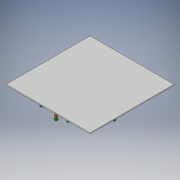
# Autodesk Inventor part: parker
Saved by Autodesk Inventor 2018 (Build 220112000, 112)
## iProperties
Created: 2018-06-06
Part Number: parker
Material: Generic
Document SubType Name: Modeling
Designer: 3400746
Density: 1 g/cm^3
Appearance: Default
Author: 3400746
Autodesk Inventor part; units mm, degrees
sketch "Sketch1" plane through (0, 0, 0) normal (0, 1, 0) x (-1, 0, 0)
  line L0 (0, 0) -> (-2159, 0)
  line L1 (-2159, 0) -> (-2159, 2159)
  line L2 (-2159, 2159) -> (0, 2159)
  line L3 (0, 2159) -> (0, 0)
  dimension "d0" = 2159
  dimension "d1" = 2159
  dimension "d2" = 2159
  constraints: 8 end point, 2 perpendicular, 1 horizontal
  measures "d0" distance of L0.start L0.end
  measures "d1" distance of L0.end L1.end
  measures "d2" distance of L1.end L2.end
extrude "Extrusion1" add sketch "Sketch1" against normal blind 25.4
sketch "Sketch2" plane through (0, -25.4, 0) normal (0, -1, 0) x (1, 0, 0)
  line L0 (0, 0) -> (0, 1079.5)
  line L1 (0, 2159) -> (0, 0) projected
  line L2 (0, 1079.5) -> (0, 1016)
  line L3 (0, 1079.5) -> (0, 1143)
  line L4 (2159, 0) -> (2159, 2159) projected
  line L5 (0, 0) -> (2159, 0) projected
  line L6 (0, 0) -> (1079.5, 0)
  line L7 (1079.5, 0) -> (1143, 0)
  line L8 (1079.5, 0) -> (1016, 0)
  line L9 (0, 1016) -> (1016, 1016)
  line L10 (1016, 0) -> (1016, 1016)
  line L11 (1016, 0) -> (1143, 0)
  line L12 (1143, 0) -> (1143, 1016)
  line L13 (1143, 1016) -> (2159, 1016)
  line L14 (2159, 1016) -> (2159, 1143)
  line L15 (2159, 1143) -> (1143, 1143)
  line L16 (1143, 1143) -> (1143, 2159)
  line L17 (1143, 2159) -> (1016, 2159)
  line L18 (2159, 2159) -> (0, 2159) projected
  line L19 (1016, 2159) -> (1016, 1143)
  line L20 (1016, 1143) -> (0, 1143)
  line L21 (0, 1143) -> (0, 1016)
  dimension "d5" = 63.5
  dimension "d6" = 63.5
  dimension "d7" = 1079.5
  dimension "d8" = 63.5
  dimension "d9" = 63.5
  constraints: 36 end point, 6 point on line, 3 perpendicular, 2 collinear, 1 midpoint
  measures "d5" distance of L0.end L2.end
  measures "d6" distance of L0.end L3.end
  measures "d7" distance of L0.start L6.end
  measures "d8" distance of L6.end L7.end
  measures "d9" distance of L6.end L8.end
extrude "Extrusion2" add sketch "Sketch2" along normal blind 2.54 contours L0 L1 L20 L19 L17 L16 L15 L4 L13 L12 L5 L10 L9
sketch "Sketch3" plane through (0, -25.4, 0) normal (0, -1, 0) x (1, 0, 0)
  line L0 (0, 2159) -> (0, 0) projected
  line L1 (0, 0) -> (0, 539.75)
  line L2 (0, 539.75) -> (508, 539.75)
  line L3 (508, 539.75) -> (508, 0)
  line L4 (508, 539.75) -> (508, 777.875)
  line L5 (508, 777.875) -> (762, 777.875)
  circle A0 centre (762, 777.875) radius 38.1
  line L6 (508, 269.875) -> (254, 269.875)
  circle A1 centre (254, 269.875) radius 35.56
  line L7 (508, 539.75) -> (818.4812, 539.75)
  circle A2 centre (818.4812, 539.75) radius 25.4
  line L8 (64.4175, 539.75) -> (64.4175, 939.7377)
  circle A3 centre (64.4175, 939.7377) radius 31.75
  line L9 (508, 115.5726) -> (863.9524, 246.3022)
  circle A4 centre (863.9524, 246.3022) radius 29.21
  line L10 (316.4036, 539.75) -> (286.0895, 847.725)
  circle A5 centre (286.0895, 847.725) radius 25.4
  line L11 (508, 539.75) -> (557.9761, 607.8668)
  circle A6 centre (557.9761, 607.8668) radius 31.75
  line L12 (2158.5018, 0) -> (1618.7518, 0)
  line L13 (1618.7518, 0) -> (1618.7518, 508)
  line L14 (1618.7518, 508) -> (2158.5018, 508)
  line L15 (1618.7518, 508) -> (1380.6268, 508)
  circle A7 centre (1380.6268, 762) radius 38.1
  line L16 (1888.6268, 508) -> (1888.6268, 254)
  circle A8 centre (1888.6268, 254) radius 35.56
  circle A9 centre (1618.7518, 818.4812) radius 25.4
  line L17 (1618.7518, 64.4175) -> (1218.7641, 64.4175)
  circle A10 centre (1218.7641, 64.4175) radius 31.75
  line L18 (2042.9293, 508) -> (1912.1996, 863.9524)
  circle A11 centre (1912.1996, 863.9524) radius 29.21
  line L19 (1618.7518, 316.4036) -> (1310.7768, 286.0895)
  circle A12 centre (1310.7768, 286.0895) radius 25.4
  circle A13 centre (1550.635, 557.9761) radius 31.75
  line L20 (0, 1146.7792) -> (0, 1686.5292)
  line L21 (472.4708, 1146.7792) -> (472.4708, 1654.7792)
  line L22 (472.4708, 1654.7792) -> (1012.2208, 1654.7792)
  line L23 (472.4708, 1654.7792) -> (234.3458, 1654.7792)
  circle A14 centre (234.3458, 1908.7792) radius 38.1
  line L24 (742.3458, 1654.7792) -> (742.3458, 1400.7792)
  circle A15 centre (742.3458, 1400.7792) radius 35.56
  circle A16 centre (472.4708, 1965.2604) radius 25.4
  line L25 (472.4708, 1211.1967) -> (72.4831, 1211.1967)
  circle A17 centre (72.4831, 1211.1967) radius 31.75
  line L26 (896.6483, 1654.7792) -> (765.9186, 2010.7316)
  circle A18 centre (765.9186, 2010.7316) radius 29.21
  line L27 (472.4708, 1463.1828) -> (164.4958, 1432.8687)
  circle A19 centre (164.4958, 1432.8687) radius 25.4
  circle A20 centre (404.354, 1704.7553) radius 31.75
  line L28 (1145.3553, 1146.7792) -> (1145.3553, 1686.5292)
  line L29 (1145.3553, 1686.5292) -> (1653.3553, 1686.5292)
  line L30 (1653.3553, 1686.5292) -> (1653.3553, 1146.7792)
  line L31 (1653.3553, 1686.5292) -> (1653.3553, 1924.6542)
  circle A21 centre (1907.3553, 1924.6542) radius 38.1
  line L32 (1653.3553, 1416.6542) -> (1399.3553, 1416.6542)
  circle A22 centre (1399.3553, 1416.6542) radius 35.56
  circle A23 centre (1963.8365, 1686.5292) radius 25.4
  line L33 (1209.7728, 1686.5292) -> (1209.7728, 2086.5169)
  circle A24 centre (1209.7728, 2086.5169) radius 31.75
  line L34 (1653.3553, 1262.3517) -> (2009.3077, 1393.0814)
  circle A25 centre (2009.3077, 1393.0814) radius 29.21
  line L35 (1461.7589, 1686.5292) -> (1431.4448, 1994.5042)
  circle A26 centre (1431.4448, 1994.5042) radius 25.4
  circle A27 centre (1703.3314, 1754.646) radius 31.75
  dimension "d12" = 539.75
  dimension "d13" = 508
  dimension "d14" = 238.125
  dimension "d15" = 254
  dimension "d16" = 76.2
  dimension "d17" = 254
  dimension "d18" = 71.12
  dimension "d19" = 50.8
  dimension "d20" = 63.5
  dimension "d21" = 58.42
  dimension "d22" = 50.8
  dimension "d67" = 63.5
  dimension "d74" = 539.75
  dimension "d75" = 508
  dimension "d76" = 238.125
  dimension "d77" = 76.2
  dimension "d78" = 254
  dimension "d79" = 71.12
  dimension "d80" = 50.8
  dimension "d81" = 63.5
  dimension "d82" = 58.42
  dimension "d83" = 50.8
  dimension "d84" = 63.5
  dimension "d85" = 539.75
  dimension "d86" = 508
  dimension "d87" = 238.125
  dimension "d88" = 76.2
  dimension "d89" = 254
  dimension "d90" = 71.12
  dimension "d91" = 50.8
  dimension "d92" = 63.5
  dimension "d93" = 58.42
  dimension "d94" = 50.8
  dimension "d95" = 63.5
  dimension "d96" = 539.75
  dimension "d97" = 508
  dimension "d98" = 238.125
  dimension "d99" = 76.2
  dimension "d100" = 254
  dimension "d101" = 71.12
  dimension "d102" = 50.8
  dimension "d103" = 63.5
  dimension "d104" = 58.42
  dimension "d105" = 50.8
  dimension "d106" = 63.5
  constraints: 70 end point, 28 centre point, 19 coincident, 13 point on line, 8 perpendicular, 4 midpoint, 4 vertical, 3 horizontal
  measures "d12" distance of L0.end L1.end
  measures "d13" distance of L1.end L2.end
  measures "d14" distance of L2.end L4.end
  measures "d15" distance of L4.end L5.end
  measures "d16" diameter of A0
  measures "d17" distance of L6.start L6.end
  measures "d18" diameter of A1
  measures "d19" diameter of A2
  measures "d20" diameter of A3
  measures "d21" diameter of A4
  measures "d22" diameter of A5
  measures "d67" diameter of A6
  measures "d74" distance of L12.start L13.start
  measures "d75" distance of L13.start L13.end
  measures "d76" distance of L13.end L15.end
  measures "d77" diameter of A7
  measures "d78" distance of L16.start L16.end
  measures "d79" diameter of A8
  measures "d80" diameter of A9
  measures "d81" diameter of A10
  measures "d82" diameter of A11
  measures "d83" diameter of A12
  measures "d84" diameter of A13
  measures "d85" distance of L20.end L20.start
  measures "d86" distance of L21.start L21.end
  measures "d87" distance of L21.end L23.end
  measures "d88" diameter of A14
  measures "d89" distance of L24.start L24.end
  measures "d90" diameter of A15
  measures "d91" diameter of A16
  measures "d92" diameter of A17
  measures "d93" diameter of A18
  measures "d94" diameter of A19
  measures "d95" diameter of A20
  measures "d96" distance of L28.start L29.start
  measures "d97" distance of L29.start L29.end
  measures "d98" distance of L29.end L31.end
  measures "d99" diameter of A21
  measures "d100" distance of L32.start L32.end
  measures "d101" diameter of A22
  measures "d102" diameter of A23
  measures "d103" diameter of A24
  measures "d104" diameter of A25
  measures "d105" diameter of A26
  measures "d106" diameter of A27
extrude "Extrusion5" add sketch "Sketch3" along normal blind 127 contours A0
extrude "Extrusion6" add sketch "Sketch3" along normal blind 152.4 contours A2
extrude "Extrusion7" add sketch "Sketch3" along normal blind 127 contours A4
extrude "Extrusion8" add sketch "Sketch3" along normal blind 165.1 contours A1
extrude "Extrusion9" add sketch "Sketch3" along normal blind 152.4 contours A5
extrude "Extrusion10" add sketch "Sketch3" along normal blind 177.8 contours A3
ref_plane "Work Plane1" through (64.4175, -203.2, 907.9877) normal (1, 0, 0) x (0, 0, 1)
sketch "Sketch10" plane through (64.4175, -203.2, 907.9877) normal (1, 0, 0) x (0, 0, 1)
  line L0 (63.5, 0) -> (0, 0) projected
  line L1 (31.75, 0) -> (31.75, 50.9666)
  line L2 (31.75, 0) -> (31.75, -50.9778)
  arc A0 (31.75, 50.9666) -> (31.75, -50.9778) centre (16.1162, -0.0056) ccw
  point P0 (-907.9877, -203.2)
  dimension "d41" = 50.9778
  constraints: 4 end point, 2 point on circle, 2 vertical, 1 centre point, 1 midpoint
  measures "d41" distance of L1.start L2.end
sketch "Sketch11" plane through (286.0895, -177.8, 847.725) normal (0, -1, 0) x (1, 0, 0)
  line L0 (0, 0) -> (0, -25.4)
  circle A0 centre (0, 0) radius 25.4 projected
  point P0 (-286.0895, -847.725)
  constraints: 2 end point, 1 vertical, 1 vertical alignment, 1 other
ref_plane "Work Plane2" through (286.0895, -177.8, 847.725) normal (-1, 0, 0) x (0, 0, -1)
sketch "Sketch12" plane through (286.0895, -177.8, 847.725) normal (-1, 0, 0) x (0, 0, -1)
  line L0 (25.4, 0) -> (-25.4, 0) projected
  line L1 (0, 0) -> (0, 45.72)
  line L2 (0, 0) -> (0, -45.72)
  arc A0 (0, -45.72) -> (0, 45.72) centre (5.3528, 0) ccw
  point P0 (847.725, -177.8)
  dimension "d44" = 45.72
  dimension "d45" = 45.72
  constraints: 4 end point, 2 point on circle, 2 vertical, 1 centre point, 1 midpoint
  measures "d44" distance of L1.start L1.end
  measures "d45" distance of L1.start L2.end
revolve "Revolution2" add sketch "Sketch12" angle 360 about axis through (286.0895, -177.8, 847.725) along (0, -1, 0)
revolve "Revolution3" add sketch "Sketch10" angle 360 about axis through (64.4175, -203.2, 939.7377) along (0, -1, 0)
sketch "Sketch13" plane through (762, -152.4, 777.875) normal (0, -1, 0) x (1, 0, 0)
  line L0 (0, 0) -> (0, -38.1)
  circle A0 centre (0, 0) radius 38.1 projected
  point P0 (-762, -777.875)
  constraints: 2 end point, 1 vertical, 1 vertical alignment, 1 other
ref_plane "Work Plane3" through (762, -152.4, 777.875) normal (-1, 0, 0) x (0, 0, -1)
sketch "Sketch14" plane through (762, -152.4, 777.875) normal (-1, 0, 0) x (0, 0, -1)
  line L0 (38.1, 0) -> (-38.1, 0) projected
  line L1 (0, 0) -> (0, 53.34)
  line L2 (0, 0) -> (0, -53.34)
  arc A0 (0, -53.34) -> (0, 53.34) centre (4.894, 0) ccw
  point P0 (777.875, -152.4)
  dimension "d49" = 53.34
  dimension "d50" = 53.34
  constraints: 4 end point, 2 point on circle, 2 vertical, 1 centre point, 1 midpoint
  measures "d49" distance of L1.start L1.end
  measures "d50" distance of L1.start L2.end
revolve "Revolution4" add sketch "Sketch14" angle 360 about axis through (762, -152.4, 777.875) along (0, -1, 0)
sketch "Sketch15" plane through (818.4812, -177.8, 539.75) normal (0, -1, 0) x (1, 0, 0)
  line L0 (0, 0) -> (0, -25.4)
  circle A0 centre (0, 0) radius 25.4 projected
  point P0 (-818.4812, -539.75)
  constraints: 2 end point, 1 vertical, 1 vertical alignment, 1 other
ref_plane "Work Plane4" through (818.4812, -177.8, 539.75) normal (-1, 0, 0) x (0, 0, -1)
sketch "Sketch17" plane through (818.4812, -177.8, 539.75) normal (-1, 0, 0) x (0, 0, -1)
  line L0 (25.4, 0) -> (-25.4, 0) projected
  line L1 (0, 0) -> (0, 43.18)
  line L2 (0, 0) -> (0, -43.18)
  arc A0 (0, -43.18) -> (0, 43.18) centre (-0.7299, 0) ccw
  point P0 (539.75, -177.8)
  dimension "d53" = 43.18
  dimension "d54" = 43.18
  constraints: 4 end point, 2 point on circle, 2 vertical, 1 centre point, 1 midpoint
  measures "d53" distance of L1.start L1.end
  measures "d54" distance of L1.start L2.end
revolve "Revolution5" add sketch "Sketch17" angle 360 about axis through (818.4812, -177.8, 539.75) along (0, -1, 0)
sketch "Sketch18" plane through (863.9524, -152.4, 246.3022) normal (0, -1, 0) x (1, 0, 0)
  circle A0 centre (0, 0) radius 29.21 projected
  line L0 (0, 0) -> (0, -29.21)
  point P0 (-863.9524, -246.3022)
  constraints: 2 end point, 1 vertical, 1 vertical alignment, 1 other
ref_plane "Work Plane5" through (863.9524, -152.4, 246.3022) normal (-1, 0, 0) x (0, 0, -1)
sketch "Sketch19" plane through (863.9524, -152.4, 246.3022) normal (-1, 0, 0) x (0, 0, -1)
  line L0 (29.21, 0) -> (-29.21, 0) projected
  line L1 (0, 0) -> (0, 38.1)
  line L2 (0, 0) -> (0, -38.1)
  arc A0 (0, -38.1) -> (0, 38.1) centre (14.1421, 0) ccw
  point P0 (246.3022, -152.4)
  dimension "d57" = 38.1
  dimension "d58" = 38.1
  dimension "d59" = 40.64
  constraints: 4 end point, 2 point on circle, 2 vertical, 1 centre point, 1 midpoint
  measures "d57" distance of L1.start L1.end
  measures "d58" distance of L1.start L2.end
  measures "d59" radius of A0
revolve "Revolution6" add sketch "Sketch19" angle 360 about axis through (863.9524, -152.4, 246.3022) along (0, -1, 0)
sketch "Sketch20" plane through (254, -190.5, 269.875) normal (0, -1, 0) x (1, 0, 0)
  line L0 (0, 0) -> (0, -35.56)
  circle A0 centre (0, 0) radius 35.56 projected
  point P0 (-254, -269.875)
  constraints: 2 end point, 1 vertical, 1 vertical alignment, 1 other
ref_plane "Work Plane6" through (254, -190.5, 269.875) normal (-1, 0, 0) x (0, 0, -1)
sketch "Sketch21" plane through (254, -190.5, 269.875) normal (-1, 0, 0) x (0, 0, -1)
  line L0 (35.56, 0) -> (-35.56, 0) projected
  line L1 (0, 0) -> (0, 55.88)
  line L2 (0, 0) -> (0, -55.88)
  arc A0 (0, -55.88) -> (0, 55.88) centre (11.9812, 0) ccw
  point P0 (269.875, -190.5)
  dimension "d63" = 55.88
  dimension "d64" = 55.88
  dimension "d65" = 57.15
  constraints: 4 end point, 2 point on circle, 2 vertical, 1 centre point, 1 midpoint
  measures "d63" distance of L1.start L1.end
  measures "d64" distance of L1.start L2.end
  measures "d65" radius of A0
revolve "Revolution7" add sketch "Sketch21" angle 360 about axis through (254, -190.5, 269.875) along (0, -1, 0)
extrude "Extrusion11" add sketch "Sketch3" along normal blind 139.7 contours A6
sketch "Sketch22" plane through (557.9761, -165.1, 607.8668) normal (0, -1, 0) x (1, 0, 0)
  line L0 (0, 0) -> (0, -31.75)
  circle A0 centre (0, 0) radius 31.75 projected
  point P0 (-557.9761, -607.8668)
  constraints: 2 end point, 1 vertical, 1 vertical alignment, 1 other
ref_plane "Work Plane7" through (557.9761, -165.1, 607.8668) normal (-1, 0, 0) x (0, 0, -1)
sketch "Sketch23" plane through (557.9761, -165.1, 607.8668) normal (-1, 0, 0) x (0, 0, -1)
  line L0 (31.75, 0) -> (-31.75, 0) projected
  line L1 (0, 0) -> (0, 48.26)
  line L2 (0, 0) -> (0, -48.26)
  arc A0 (0, -48.26) -> (0, 48.26) centre (-0.8159, 0) ccw
  point P0 (607.8668, -165.1)
  dimension "d71" = 48.26
  dimension "d72" = 48.26
  constraints: 4 end point, 2 point on circle, 2 vertical, 1 centre point, 1 midpoint
  measures "d71" distance of L1.start L1.end
  measures "d72" distance of L1.start L2.end
revolve "Revolution8" add sketch "Sketch23" angle 360 about axis through (557.9761, -165.1, 607.8668) along (0, -1, 0)
extrude "Extrusion12" add sketch "Sketch3" along normal blind 127 contours A7 | A15 | A22
sketch "Sketch24" plane through (1399.3553, -152.4, 1416.6542) normal (0, -1, 0) x (1, 0, 0)
  line L0 (0, 0) -> (0, -35.56)
  circle A0 centre (0, 0) radius 35.56 projected
  point P0 (-1399.3553, -1416.6542)
  constraints: 2 end point, 1 vertical, 1 vertical alignment, 1 other
ref_plane "Work Plane8" through (1399.3553, -152.4, 1416.6542) normal (-1, 0, 0) x (0, 0, -1)
sketch "Sketch25" plane through (1399.3553, -152.4, 1416.6542) normal (-1, 0, 0) x (0, 0, -1)
  line L0 (0, 0) -> (0, 50.8)
  line L1 (0, 0) -> (0, -50.8)
  arc A0 (0, -50.8) -> (0, 50.8) centre (0, 0) ccw
  point P0 (1416.6542, -152.4)
  dimension "d110" = 50.8
  dimension "d111" = 50.8
  dimension "d112" = 50.8
  constraints: 4 end point, 2 point on circle, 2 vertical, 1 centre point
  measures "d110" distance of L0.start L0.end
  measures "d111" distance of L0.start L1.end
  measures "d112" radius of A0
revolve "Revolution9" add sketch "Sketch25" angle 360 about axis through (1399.3553, -152.4, 1416.6542) along (0, -1, 0)
sketch "Sketch26" plane through (1380.6268, -152.4, 762) normal (0, -1, 0) x (1, 0, 0)
  line L0 (0, 0) -> (0, -38.1)
  circle A0 centre (0, 0) radius 38.1 projected
  point P0 (-1380.6268, -762)
  constraints: 2 end point, 1 vertical, 1 vertical alignment, 1 other
ref_plane "Work Plane9" through (1380.6268, -152.4, 762) normal (-1, 0, 0) x (0, 0, -1)
sketch "Sketch27" plane through (1380.6268, -152.4, 762) normal (-1, 0, 0) x (0, 0, -1)
  line L0 (38.1, 0) -> (-38.1, 0) projected
  line L1 (0, 0) -> (0, 50.8)
  line L2 (0, 0) -> (0, -50.8)
  arc A0 (0, -50.8) -> (0, 50.8) centre (0, 0) ccw
  point P0 (762, -152.4)
  dimension "d115" = 50.8
  dimension "d116" = 50.8
  dimension "d117" = 50.8
  constraints: 4 end point, 2 point on circle, 2 vertical, 1 centre point, 1 midpoint
  measures "d115" distance of L1.start L1.end
  measures "d116" distance of L1.start L2.end
  measures "d117" radius of A0
revolve "Revolution10" add sketch "Sketch27" angle 360 about axis through (1380.6268, -152.4, 762) along (0, -1, 0)
sketch "Sketch28" plane through (742.3458, -152.4, 1400.7792) normal (0, -1, 0) x (1, 0, 0)
  circle A0 centre (0, 0) radius 35.56 projected
  line L0 (0, 0) -> (0, -35.56)
  point P0 (-742.3458, -1400.7792)
  constraints: 2 end point, 1 vertical, 1 vertical alignment, 1 other
ref_plane "Work Plane10" through (742.3458, -152.4, 1400.7792) normal (-1, 0, 0) x (0, 0, -1)
sketch "Sketch29" plane through (742.3458, -152.4, 1400.7792) normal (-1, 0, 0) x (0, 0, -1)
  line L0 (0, 0) -> (0, 50.8)
  line L1 (0, 0) -> (0, -50.8)
  arc A0 (0, -50.8) -> (0, 50.8) centre (0, 0) ccw
  point P0 (1400.7792, -152.4)
  dimension "d120" = 50.8
  dimension "d121" = 50.8
  dimension "d122" = 50.8
  constraints: 4 end point, 2 point on circle, 2 vertical, 1 centre point
  measures "d120" distance of L0.start L0.end
  measures "d121" distance of L0.start L1.end
  measures "d122" radius of A0
revolve "Revolution11" add sketch "Sketch29" angle 360 about axis through (742.3458, -152.4, 1400.7792) along (0, -1, 0)
extrude "Extrusion13" add sketch "Sketch3" along normal blind 127 contours A11 | A18 | A25
sketch "Sketch30" plane through (765.9186, -152.4, 2010.7316) normal (0, -1, 0) x (1, 0, 0)
  circle A0 centre (0, 0) radius 29.21 projected
  line L0 (0, 0) -> (0, -38.1)
  point P0 (-765.9186, -2010.7316)
  dimension "d126" = 38.1
  constraints: 2 end point, 1 vertical
  measures "d126" distance of L0.start L0.end
ref_plane "Work Plane11" through (765.9186, -152.4, 2010.7316) normal (-1, 0, 0) x (0, 0, -1)
sketch "Sketch31" plane through (765.9186, -152.4, 2010.7316) normal (-1, 0, 0) x (0, 0, -1)
  line L0 (0, 0) -> (0, 45.72)
  line L1 (0, 0) -> (0, -45.72)
  arc A0 (0, -45.72) -> (0, 45.72) centre (0, 0) ccw
  point P0 (2010.7316, -152.4)
  dimension "d128" = 45.72
  dimension "d129" = 45.72
  dimension "d130" = 45.72
  constraints: 4 end point, 2 point on circle, 2 vertical, 1 centre point
  measures "d128" distance of L0.start L0.end
  measures "d129" distance of L0.start L1.end
  measures "d130" radius of A0
revolve "Revolution12" add sketch "Sketch31" angle 360 about axis through (765.9186, -152.4, 2010.7316) along (0, -1, 0)
sketch "Sketch32" plane through (2009.3077, -152.4, 1393.0814) normal (0, -1, 0) x (1, 0, 0)
  line L0 (0, 0) -> (0, -29.21)
  circle A0 centre (0, 0) radius 29.21 projected
  point P0 (-2009.3077, -1393.0814)
  constraints: 2 end point, 1 vertical, 1 vertical alignment, 1 other
ref_plane "Work Plane12" through (2009.3077, -152.4, 1393.0814) normal (-1, 0, 0) x (0, 0, -1)
sketch "Sketch33" plane through (2009.3077, -152.4, 1393.0814) normal (-1, 0, 0) x (0, 0, -1)
  line L0 (0, 0) -> (0, 45.72)
  line L1 (0, 0) -> (0, -45.72)
  arc A0 (0, -45.72) -> (0, 45.72) centre (0, 0) ccw
  point P0 (1393.0814, -152.4)
  dimension "d133" = 45.72
  dimension "d134" = 45.72
  dimension "d135" = 45.72
  constraints: 4 end point, 2 point on circle, 2 vertical, 1 centre point
  measures "d133" distance of L0.start L0.end
  measures "d134" distance of L0.start L1.end
  measures "d135" radius of A0
revolve "Revolution13" add sketch "Sketch33" angle 360 about axis through (2009.3077, -152.4, 1393.0814) along (0, -1, 0)
sketch "Sketch34" plane through (1912.1996, -152.4, 863.9524) normal (0, -1, 0) x (1, 0, 0)
  line L0 (0, 0) -> (0, -29.21)
  circle A0 centre (0, 0) radius 29.21 projected
  point P0 (-1912.1996, -863.9524)
  constraints: 2 end point, 1 vertical, 1 vertical alignment, 1 other
ref_plane "Work Plane13" through (1912.1996, -152.4, 863.9524) normal (-1, 0, 0) x (0, 0, -1)
sketch "Sketch35" plane through (1912.1996, -152.4, 863.9524) normal (-1, 0, 0) x (0, 0, -1)
  line L0 (0, 0) -> (0, 45.72)
  line L1 (0, 0) -> (0, -45.72)
  arc A0 (0, -45.72) -> (0, 45.72) centre (0, 0) ccw
  point P0 (863.9524, -152.4)
  dimension "d138" = 45.72
  dimension "d140" = 45.72
  dimension "d141" = 45.72
  constraints: 4 end point, 2 point on circle, 2 vertical, 1 centre point
  measures "d138" distance of L0.start L0.end
  measures "d140" distance of L0.start L1.end
  measures "d141" radius of A0
revolve "Revolution14" add sketch "Sketch35" angle 360 about axis through (1912.1996, -152.4, 863.9524) along (0, -1, 0)
extrude "Extrusion14" add sketch "Sketch3" along normal blind 152.4 contours A9 | A12 | A16 | A19 | A23 | A26
sketch "Sketch36" plane through (472.4708, -177.8, 1965.2604) normal (0, -1, 0) x (1, 0, 0)
  circle A0 centre (0, 0) radius 25.4 projected
  line L0 (0, 0) -> (0, -25.4)
  point P0 (-472.4708, -1965.2604)
  constraints: 2 end point, 1 vertical, 1 vertical alignment, 1 other
ref_plane "Work Plane14" through (472.4708, -177.8, 1965.2604) normal (-1, 0, 0) x (0, 0, -1)
sketch "Sketch37" plane through (472.4708, -177.8, 1965.2604) normal (-1, 0, 0) x (0, 0, -1)
  line L0 (0, 0) -> (0, 38.1)
  line L1 (0, 0) -> (0, -38.1)
  arc A0 (0, -38.1) -> (0, 38.1) centre (0, 0) ccw
  point P0 (1965.2604, -177.8)
  dimension "d146" = 38.1
  dimension "d147" = 38.1
  dimension "d148" = 38.1
  constraints: 4 end point, 2 point on circle, 2 vertical, 1 centre point
  measures "d146" distance of L0.start L0.end
  measures "d147" distance of L0.start L1.end
  measures "d148" radius of A0
revolve "Revolution15" add sketch "Sketch37" angle 360 about axis through (472.4708, -177.8, 1965.2604) along (0, -1, 0)
sketch "Sketch38" plane through (164.4958, -177.8, 1432.8687) normal (0, -1, 0) x (1, 0, 0)
  circle A0 centre (0, 0) radius 25.4 projected
  line L0 (0, 0) -> (0, -25.4)
  point P0 (-164.4958, -1432.8687)
  constraints: 2 end point, 1 vertical, 1 vertical alignment, 1 other
ref_plane "Work Plane15" through (164.4958, -177.8, 1432.8687) normal (-1, 0, 0) x (0, 0, -1)
sketch "Sketch39" plane through (164.4958, -177.8, 1432.8687) normal (-1, 0, 0) x (0, 0, -1)
  line L0 (25.4, 0) -> (-25.4, 0) projected
  line L1 (0, 0) -> (0, 38.1)
  line L2 (0, 0) -> (0, -38.1)
  arc A0 (0, -38.1) -> (0, 38.1) centre (0, 0) ccw
  point P0 (1432.8687, -177.8)
  dimension "d151" = 38.1
  dimension "d152" = 38.1
  dimension "d153" = 38.1
  constraints: 4 end point, 2 point on circle, 2 vertical, 1 centre point, 1 midpoint
  measures "d151" distance of L1.start L1.end
  measures "d152" distance of L1.start L2.end
  measures "d153" radius of A0
revolve "Revolution16" add sketch "Sketch39" angle 360 about axis through (164.4958, -177.8, 1432.8687) along (0, -1, 0)
sketch "Sketch40" plane through (1431.4448, -177.8, 1994.5042) normal (0, -1, 0) x (1, 0, 0)
  line L0 (0, 0) -> (0, -25.5263)
  point P0 (-1431.4448, -1994.5042)
  constraints: 2 end point, 1 vertical
ref_plane "Work Plane16" through (1431.4448, -177.8, 1994.5042) normal (-1, 0, 0) x (0, 0, -1)
sketch "Sketch41" plane through (1431.4448, -177.8, 1994.5042) normal (-1, 0, 0) x (0, 0, -1)
  line L0 (0, 0) -> (0, 38.1)
  line L1 (0, 0) -> (0, -38.1)
  arc A0 (0, -38.1) -> (0, 38.1) centre (0, 0) ccw
  point P0 (1994.5042, -177.8)
  dimension "d156" = 38.1
  dimension "d158" = 38.1
  dimension "d159" = 38.1
  constraints: 4 end point, 2 point on circle, 1 centre point, 1 point on line, 1 vertical
  measures "d156" distance of L0.start L0.end
  measures "d158" distance of L0.start L1.end
  measures "d159" radius of A0
revolve "Revolution17" add sketch "Sketch41" angle 360 about axis through (1431.4448, -177.8, 1994.5042) along (0, -1, 0)
sketch "Sketch42" plane through (1963.8365, -177.8, 1686.5292) normal (0, -1, 0) x (1, 0, 0)
  line L0 (0, 0) -> (0, -25.4)
  circle A0 centre (0, 0) radius 25.4 projected
  point P0 (-1963.8365, -1686.5292)
  constraints: 2 end point, 1 vertical, 1 vertical alignment, 1 other
ref_plane "Work Plane17" through (1963.8365, -177.8, 1686.5292) normal (-1, 0, 0) x (0, 0, -1)
sketch "Sketch43" plane through (1963.8365, -177.8, 1686.5292) normal (-1, 0, 0) x (0, 0, -1)
  line L0 (25.4, 0) -> (-25.4, 0) projected
  line L1 (0, 0) -> (0, 38.1)
  line L2 (0, 0) -> (0, -38.1)
  arc A0 (0, -38.1) -> (0, 38.1) centre (0, 0) ccw
  point P0 (1686.5292, -177.8)
  dimension "d162" = 38.1
  dimension "d163" = 38.1
  dimension "d164" = 38.1
  constraints: 4 end point, 2 point on circle, 2 vertical, 1 centre point, 1 midpoint
  measures "d162" distance of L1.start L1.end
  measures "d163" distance of L1.start L2.end
  measures "d164" radius of A0
revolve "Revolution18" add sketch "Sketch43" angle 360 about axis through (1963.8365, -177.8, 1686.5292) along (0, -1, 0)
sketch "Sketch44" plane through (1618.7518, -177.8, 818.4812) normal (0, -1, 0) x (1, 0, 0)
  line L0 (0, 0) -> (0, -25.4)
  circle A0 centre (0, 0) radius 25.4 projected
  point P0 (-1618.7518, -818.4812)
  constraints: 2 end point, 1 vertical, 1 vertical alignment, 1 other
ref_plane "Work Plane18" through (1618.7518, -177.8, 818.4812) normal (-1, 0, 0) x (0, 0, -1)
sketch "Sketch45" plane through (1618.7518, -177.8, 818.4812) normal (-1, 0, 0) x (0, 0, -1)
  line L0 (25.4, 0) -> (-25.4, 0) projected
  line L1 (0, 0) -> (25.4, 0)
  line L2 (0, 0) -> (0, 38.1)
  line L3 (0, 0) -> (0, -38.1)
  line L4 (0, 0) -> (38.1, 0) construction
  arc A0 (0, -38.1) -> (0, 38.1) centre (0, 0) ccw
  point P0 (818.4812, -177.8)
  dimension "d167" = 38.1
  dimension "d168" = 38.1
  dimension "d169" = 90
  dimension "d170" = 38.1
  constraints: 8 end point, 2 point on circle, 2 vertical, 1 centre point, 1 collinear, 1 horizontal, 1 midpoint, 1 perpendicular
  measures "d167" distance of L1.start L2.end
  measures "d168" distance of L1.start L3.end
  measures "d169" angle of L3 L4
  measures "d170" radius of A0
revolve "Revolution19" add sketch "Sketch45" angle 360 about axis through (1618.7518, -177.8, 818.4812) along (0, -1, 0)
sketch "Sketch46" plane through (1310.7768, -177.8, 286.0895) normal (0, -1, 0) x (1, 0, 0)
  line L0 (0, 0) -> (0, -25.4)
  circle A0 centre (0, 0) radius 25.4 projected
  point P0 (-1310.7768, -286.0895)
  constraints: 2 end point, 1 vertical, 1 vertical alignment, 1 other
ref_plane "Work Plane19" through (1310.7768, -177.8, 286.0895) normal (-1, 0, 0) x (0, 0, -1)
sketch "Sketch47" plane through (1310.7768, -177.8, 286.0895) normal (-1, 0, 0) x (0, 0, -1)
  line L0 (0, 0) -> (0, 38.1)
  line L1 (0, 0) -> (0, -38.1)
  line L2 (0, 0) -> (38.1, 0) construction
  arc A0 (0, -38.1) -> (0, 38.1) centre (0, 0) ccw
  point P0 (286.0895, -177.8)
  dimension "d173" = 38.1
  dimension "d174" = 38.1
  dimension "d175" = 90
  dimension "d176" = 38.1
  constraints: 6 end point, 2 point on circle, 2 vertical, 1 centre point, 1 horizontal, 1 perpendicular
  measures "d173" distance of L0.start L0.end
  measures "d174" distance of L0.start L1.end
  measures "d175" angle of L1 L2
  measures "d176" radius of A0
revolve "Revolution20" add sketch "Sketch47" angle 360 about axis through (1310.7768, -177.8, 286.0895) along (0, -1, 0)
extrude "Extrusion15" add sketch "Sketch3" along normal blind 177.8 contours A10 | A17 | A24
extrude "Extrusion16" add sketch "Sketch3" along normal blind 139.7 contours A13 | A20 | A27
sketch "Sketch48" plane through (404.354, -165.1, 1704.7553) normal (0, -1, 0) x (1, 0, 0)
  line L0 (0, 0) -> (0, -31.75)
  circle A0 centre (0, 0) radius 31.75 projected
  point P0 (-404.354, -1704.7553)
  constraints: 2 end point, 1 vertical, 1 vertical alignment, 1 other
ref_plane "Work Plane20" through (404.354, -165.1, 1704.7553) normal (-1, 0, 0) x (0, 0, -1)
sketch "Sketch49" plane through (404.354, -165.1, 1704.7553) normal (-1, 0, 0) x (0, 0, -1)
  line L0 (31.75, 0) -> (-31.75, 0) projected
  line L1 (0, 0) -> (0, 48.26)
  line L2 (0, 0) -> (0, -48.26)
  arc A0 (0, -48.26) -> (0, 48.26) centre (0.1359, 0) ccw
  point P0 (1704.7553, -165.1)
  dimension "d183" = 48.26
  dimension "d184" = 48.26
  constraints: 4 end point, 2 point on circle, 2 vertical, 1 centre point, 1 midpoint
  measures "d183" distance of L1.start L1.end
  measures "d184" distance of L1.start L2.end
revolve "Revolution21" add sketch "Sketch49" angle 360 about axis through (404.354, -165.1, 1704.7553) along (0, -1, 0)
sketch "Sketch50" plane through (1703.3314, -165.1, 1754.646) normal (0, -1, 0) x (1, 0, 0)
  line L0 (0, 0) -> (0, -31.75)
  circle A0 centre (0, 0) radius 31.75 projected
  point P0 (-1703.3314, -1754.646)
  constraints: 2 end point, 1 vertical, 1 vertical alignment, 1 other
ref_plane "Work Plane21" through (1703.3314, -165.1, 1754.646) normal (-1, 0, 0) x (0, 0, -1)
sketch "Sketch51" plane through (1703.3314, -165.1, 1754.646) normal (-1, 0, 0) x (0, 0, -1)
  line L0 (0, 0) -> (0, 45.72)
  line L1 (0, 0) -> (0, -45.72)
  arc A0 (0, -45.72) -> (0, 45.72) centre (0, 0) ccw
  point P0 (1754.646, -165.1)
  dimension "d187" = 45.72
  dimension "d188" = 45.72
  dimension "d189" = 45.72
  constraints: 4 end point, 2 point on circle, 2 vertical, 1 centre point
  measures "d187" distance of L0.start L0.end
  measures "d188" distance of L0.start L1.end
  measures "d189" radius of A0
revolve "Revolution22" add sketch "Sketch51" angle 360 about axis through (1703.3314, -165.1, 1754.646) along (0, -1, 0)
sketch "Sketch52" plane through (1550.635, -165.1, 557.9761) normal (0, -1, 0) x (1, 0, 0)
  line L0 (0, 0) -> (0, -31.75)
  circle A0 centre (0, 0) radius 31.75 projected
  point P0 (-1550.635, -557.9761)
  constraints: 2 end point, 1 vertical, 1 vertical alignment, 1 other
ref_plane "Work Plane22" through (1550.635, -165.1, 557.9761) normal (-1, 0, 0) x (0, 0, -1)
sketch "Sketch53" plane through (1550.635, -165.1, 557.9761) normal (-1, 0, 0) x (0, 0, -1)
  line L0 (31.75, 0) -> (-31.75, 0) projected
  line L1 (0, 0) -> (0, 48.26)
  line L2 (0, 0) -> (0, -48.26)
  arc A0 (0, -48.26) -> (0, 48.26) centre (0, 0) ccw
  point P0 (557.9761, -165.1)
  dimension "d192" = 48.26
  dimension "d193" = 48.26
  dimension "d194" = 48.26
  constraints: 4 end point, 2 point on circle, 2 vertical, 1 centre point, 1 midpoint
  measures "d192" distance of L1.start L1.end
  measures "d193" distance of L1.start L2.end
  measures "d194" radius of A0
revolve "Revolution23" add sketch "Sketch53" angle 360 about axis through (1550.635, -165.1, 557.9761) along (0, -1, 0)
sketch "Sketch54" plane through (1218.7641, -203.2, 64.4175) normal (0, -1, 0) x (1, 0, 0)
  circle A0 centre (0, 0) radius 31.75 projected
  line L0 (0, 0) -> (0, -31.75)
  point P0 (-1218.7641, -64.4175)
  constraints: 2 end point, 1 vertical, 1 vertical alignment, 1 other
ref_plane "Work Plane23" through (1218.7641, -203.2, 64.4175) normal (-1, 0, 0) x (0, 0, -1)
sketch "Sketch55" plane through (1218.7641, -203.2, 64.4175) normal (-1, 0, 0) x (0, 0, -1)
  line L0 (0, 0) -> (0, 45.72)
  line L1 (0, 0) -> (0, -45.72)
  arc A0 (0, -45.72) -> (0, 45.72) centre (0, 0) ccw
  point P0 (64.4175, -203.2)
  dimension "d197" = 45.72
  dimension "d198" = 45.72
  dimension "d199" = 45.72
  constraints: 4 end point, 2 point on circle, 2 vertical, 1 centre point
  measures "d197" distance of L0.start L0.end
  measures "d198" distance of L0.start L1.end
  measures "d199" radius of A0
revolve "Revolution24" add sketch "Sketch55" angle 360 about axis through (1218.7641, -203.2, 64.4175) along (0, -1, 0)
extrude "Extrusion17" add sketch "Sketch3" along normal blind 165.1 contours A8 | A14 | A21
sketch "Sketch56" plane through (72.4831, -203.2, 1211.1967) normal (0, -1, 0) x (1, 0, 0)
  line L0 (0, 0) -> (0, -31.75)
  circle A0 centre (0, 0) radius 31.75 projected
  point P0 (-72.4831, -1211.1967)
  constraints: 2 end point, 1 vertical, 1 vertical alignment, 1 other
ref_plane "Work Plane24" through (72.4831, -203.2, 1211.1967) normal (-1, 0, 0) x (0, 0, -1)
sketch "Sketch57" plane through (72.4831, -203.2, 1211.1967) normal (-1, 0, 0) x (0, 0, -1)
  line L0 (0, 0) -> (40.64, 0)
  line L1 (0, 0) -> (0, -40.64)
  line L2 (0, 0) -> (0, 40.64)
  arc A0 (0, -40.64) -> (0, 40.64) centre (0, 0) ccw
  point P0 (1211.1967, -203.2)
  dimension "d205" = 40.64
  dimension "d206" = 40.64
  dimension "d207" = 40.64
  constraints: 6 end point, 2 point on circle, 2 vertical, 1 centre point
  measures "d205" distance of L0.start L1.end
  measures "d206" distance of L0.start L2.end
  measures "d207" radius of A0
revolve "Revolution25" add sketch "Sketch57" angle 360 about axis through (72.4831, -203.2, 1211.1967) along (0, -1, 0)
sketch "Sketch58" plane through (234.3458, -190.5, 1908.7792) normal (0, -1, 0) x (1, 0, 0)
  circle A0 centre (0, 0) radius 38.1 projected
  line L0 (0, 0) -> (0, -38.1)
  point P0 (-234.3458, -1908.7792)
  constraints: 2 end point, 1 vertical, 1 vertical alignment, 1 other
ref_plane "Work Plane25" through (234.3458, -190.5, 1908.7792) normal (-1, 0, 0) x (0, 0, -1)
sketch "Sketch59" plane through (234.3458, -190.5, 1908.7792) normal (-1, 0, 0) x (0, 0, -1)
  line L0 (0, 0) -> (0, 45.72)
  line L1 (0, 0) -> (0, -45.72)
  arc A0 (0, -45.72) -> (0, 45.72) centre (0, 0) ccw
  point P0 (1908.7792, -190.5)
  dimension "d210" = 45.72
  dimension "d211" = 45.72
  dimension "d212" = 45.72
  constraints: 4 end point, 2 point on circle, 2 vertical, 1 centre point
  measures "d210" distance of L0.start L0.end
  measures "d211" distance of L0.start L1.end
  measures "d212" radius of A0
revolve "Revolution26" add sketch "Sketch59" angle 360 about axis through (234.3458, -190.5, 1908.7792) along (0, -1, 0)
sketch "Sketch60" plane through (1209.7728, -203.2, 2086.5169) normal (0, -1, 0) x (1, 0, 0)
  line L0 (0, 0) -> (0, -31.75)
  circle A0 centre (0, 0) radius 31.75 projected
  point P0 (-1209.7728, -2086.5169)
  constraints: 2 end point, 1 vertical, 1 vertical alignment, 1 other
ref_plane "Work Plane26" through (1209.7728, -203.2, 2086.5169) normal (-1, 0, 0) x (0, 0, -1)
sketch "Sketch61" plane through (1209.7728, -203.2, 2086.5169) normal (-1, 0, 0) x (0, 0, -1)
  line L0 (31.75, 0) -> (-31.75, 0) projected
  line L1 (0, 0) -> (0, 43.18)
  line L2 (0, 0) -> (0, -43.18)
  arc A0 (0, -43.18) -> (0, 43.18) centre (0, 0) ccw
  point P0 (2086.5169, -203.2)
  dimension "d215" = 43.18
  dimension "d216" = 43.18
  dimension "d217" = 43.18
  constraints: 4 end point, 2 point on circle, 2 vertical, 1 centre point, 1 midpoint
  measures "d215" distance of L1.start L1.end
  measures "d216" distance of L1.start L2.end
  measures "d217" radius of A0
revolve "Revolution27" add sketch "Sketch61" angle 360 about axis through (1209.7728, -203.2, 2086.5169) along (0, -1, 0)
sketch "Sketch62" plane through (1907.3553, -190.5, 1924.6542) normal (0, -1, 0) x (1, 0, 0)
  line L0 (0, 0) -> (0, -38.1)
  circle A0 centre (0, 0) radius 38.1 projected
  point P0 (-1907.3553, -1924.6542)
  constraints: 2 end point, 1 vertical, 1 vertical alignment, 1 other
ref_plane "Work Plane27" through (1907.3553, -190.5, 1924.6542) normal (-1, 0, 0) x (0, 0, -1)
sketch "Sketch63" plane through (1907.3553, -190.5, 1924.6542) normal (-1, 0, 0) x (0, 0, -1)
  line L0 (38.1, 0) -> (-38.1, 0) projected
  line L1 (0, 0) -> (0, 48.26)
  line L2 (0, 0) -> (0, -48.26)
  arc A0 (0, -48.26) -> (0, 48.26) centre (0, 0) ccw
  point P0 (1924.6542, -190.5)
  dimension "d220" = 48.26
  dimension "d221" = 48.26
  dimension "d222" = 48.26
  constraints: 4 end point, 2 point on circle, 2 vertical, 1 centre point, 1 midpoint
  measures "d220" distance of L1.start L1.end
  measures "d221" distance of L1.start L2.end
  measures "d222" radius of A0
revolve "Revolution28" add sketch "Sketch63" angle 360 about axis through (1907.3553, -190.5, 1924.6542) along (0, -1, 0)
sketch "Sketch64" plane through (1888.6268, -190.5, 254) normal (0, -1, 0) x (1, 0, 0)
  line L0 (0, 0) -> (0, -35.56)
  circle A0 centre (0, 0) radius 35.56 projected
  point P0 (-1888.6268, -254)
  constraints: 2 end point, 1 vertical, 1 vertical alignment, 1 other
ref_plane "Work Plane28" through (1888.6268, -190.5, 254) normal (-1, 0, 0) x (0, 0, -1)
sketch "Sketch65" plane through (1888.6268, -190.5, 254) normal (-1, 0, 0) x (0, 0, -1)
  line L0 (0, 0) -> (0, 43.18)
  line L1 (0, 0) -> (0, -43.18)
  arc A0 (0, -43.18) -> (0, 43.18) centre (0, 0) ccw
  point P0 (254, -190.5)
  dimension "d225" = 43.18
  dimension "d226" = 43.18
  dimension "d227" = 43.18
  constraints: 4 end point, 2 point on circle, 2 vertical, 1 centre point
  measures "d225" distance of L0.start L0.end
  measures "d226" distance of L0.start L1.end
  measures "d227" radius of A0
revolve "Revolution29" add sketch "Sketch65" angle 360 about axis through (1888.6268, -190.5, 254) along (0, -1, 0)
body "Solid1"
